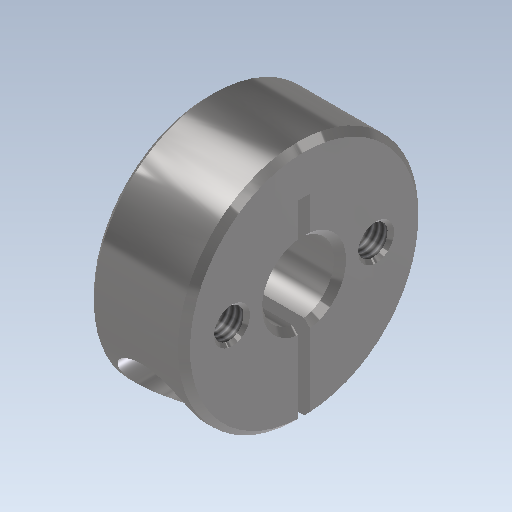
# Autodesk Inventor part: SCSW6-8b
Saved by Autodesk Inventor 2021 (Build 250183000, 183)
## iProperties
Created: 2019-10-03
Part Number: SCSW6-8b
Material: 鋼、炭素鋼
Catalog Web Link: www.cadenas.de
Description: SCSW, PSCSW, SSCSW-b-Shaft Collars - 2 Holes/2 Taps - 2-Tapped (Coarse Thread)
Vendor: MISUMI
Document SubType Name: Modeling
Designer: psadmin
Manufacturer: MISUMI
Mass: 15.1833 g
Surface Area: 15.2751 cm^2
Volume: 1.93418 cm^3
Density: 7.85 g/cm^3
Appearance: 半つや出し
Category: PARTsolutions
Company: MISUMI
PSOL_IDENT_0: {$CADENAS_DATA\23d-libs\misumi\metric\03_set_collars\scsw_b.prj},182 {VTYP=3D},{NB=SCSW6-8b},{LINA=S
PSOL_IDENT_1: CSW6-8b},{NN=SCSW, PSCSW, SSCSW-b},{DATE=30.03.2018 01:14:49},{GEOMDATE=24.02.2016 04:36:42},{VERSIO
PSOL_IDENT_2: N=},{LINEID=220},{WBVAR=MAT,ST,BS},{WBNUMERIC=BS}  {NB=SCSW6-8b},{LINA=SCSW6-8b},{KT=DUMMY},{PN=SCSW
PSOL_IDENT_3: 6-8},{TYPE=SCSW},{MAT=1045},{ST=Black Oxide},{AC=Hexagon Socket Head Set Screw 1 Pc.},{D=6},{BS=8},{
PSOL_IDENT_4: D1=20},{M=M3},{THMD=3},{THDMIN=2.459},{ST0='Black Oxide','Black Oxide','Electroless Nickel Plating','
PSOL_IDENT_5: Electroless Nickel Plating'},{B1=8,10},{DD=3.4},{R=3.00},{W=1.0},{X=6.0},{Y=4.0},{Z=6~6.5},{S=3.5},{
PSOL_IDENT_6: P=12},{C=0.5},{L=10},{M1=M3},{ZZ=6.25},{THMD1=3},{THDMIN1=2.459}
NN: SCSW, PSCSW, SSCSW-b
NT: Shaft Collars - 2 Holes/2 Taps - 2-Tapped (Coarse Thread)
NB: SCSW6-8b
NBSYN: $PN.b
LINA: SCSW6-8b
PN: SCSW6-8
MAT: S45C Equivalent
ST: Black Oxide
AC: Hexagon Socket Head Set Screw 1 Pc.
D: 6
BS: 8
D1: 20
M: M3
DD: 3.4
R: 3
W: 1
X: 6
Y: 4
Z: 6~6.5
S: 3.5
P: 12
M1: M3
SUPPLIER: MISUMI
ARTICLENO: SCSW6-8b
BOMINFO: SCSW6-8b
CREATOR: CADENAS GmbH
d17: 0.000 mm
Title: SCSW6-8b
Author: Cadenas PARTsolutions
Comments: Shaft Collars - 2 Holes/2 Taps - 2-Tapped (Coarse Thread)
Autodesk Inventor part; units mm, degrees
sketch "Sketch_1" plane through (0, 0, 0) normal (0, 0, 1) x (1, 0, 0)
  line L0 (4, 0) -> (-4, 0)
  line L1 (-4, 9.5) -> (-4, 3.5)
  line L2 (-4, 3.5) -> (-3.5, 3)
  line L3 (-3.5, 3) -> (3.5, 3)
  line L4 (3.5, 3) -> (4, 3.5)
  line L5 (4, 3.5) -> (4, 9.5)
  line L6 (4, 9.5) -> (3.5, 10)
  line L7 (3.5, 10) -> (-3.5, 10)
  line L8 (-3.5, 10) -> (-4, 9.5)
  constraints: 18 end point
revolve "Revolution1" add sketch "Sketch_1" angle 360 about axis through (4, 0, 0) along (1, 0, 0)
sketch "Sketch_2" plane through (0, 0, 0) normal (1, 0, 0) x (0, 1, 0)
  line L0 (-10, 0.5) -> (-10, -0.5)
  line L1 (-10, -0.5) -> (6.25, -0.5)
  line L2 (6.25, -0.5) -> (6.25, 0.5)
  line L3 (6.25, 0.5) -> (-10, 0.5)
  constraints: 8 end point
extrude "Extrusion1" cut sketch "Sketch_2" along normal mid plane 8
sketch "Sketch_3" plane through (0, 0, 0) normal (1, 0, 0) x (0, 1, 0)
  line L0 (-6, 10) -> (-6, 0)
  line L1 (-6, 0) -> (-7.7, 0)
  line L2 (-7.7, 0) -> (-7.7, 4)
  line L3 (-7.7, 4) -> (-9, 4)
  line L4 (-9, 4) -> (-9, 10)
  line L5 (-9, 10) -> (-6, 10)
  line L6 (-6, 10) -> (-6, 0)
  constraints: 14 end point
revolve "Revolution2" cut sketch "Sketch_3" angle 360 about axis through (0, -6, 10) along (0, 0, 1)
sketch "Sketch4" plane through (-3.5, -2.958, -0.5) normal (0, 0, 1) x (1, 0, 0)
  point P0 (3.5, -3.042)
hole "Hole1" at (0, -6, -0.5) direction (0, 0, -1) diameter 2.459 depth 9 countersink diameter 3 countersink angle 90 thread size "M3x0.5" class "6H" standard "ISO Metric profile"
sketch "Sketch_7" plane through (0, 0, -6) normal (0, 0, 1) x (1, 0, 0)
  line L0 (4, 0) -> (-4, 0)
  line L1 (-4, 0) -> (-4, 1.5)
  line L2 (-4, 1.5) -> (-3.7295, 1.2295)
  line L3 (-3.7295, 1.2295) -> (3.7295, 1.2295)
  line L4 (3.7295, 1.2295) -> (4, 1.5)
  line L5 (4, 1.5) -> (4, 0)
  line L6 (4, 0) -> (-4, 0)
  constraints: 14 end point
revolve "Revolution3" cut sketch "Sketch_7" angle 360 about axis through (4, 0, -6) along (1, 0, 0)
thread "Thread1" size "M3x0.5" class "6H" standard "ISO Metric profile" full length
sketch "Sketch_8" plane through (0, 0, 6) normal (0, 0, 1) x (1, 0, 0)
  line L0 (4, 0) -> (-4, 0)
  line L1 (-4, 0) -> (-4, 1.5)
  line L2 (-4, 1.5) -> (-3.7295, 1.2295)
  line L3 (-3.7295, 1.2295) -> (3.7295, 1.2295)
  line L4 (3.7295, 1.2295) -> (4, 1.5)
  line L5 (4, 1.5) -> (4, 0)
  line L6 (4, 0) -> (-4, 0)
  constraints: 14 end point
revolve "Revolution4" cut sketch "Sketch_8" angle 360 about axis through (4, 0, 6) along (1, 0, 0)
thread "Thread2" size "M3x0.5" class "6H" standard "ISO Metric profile" full length
ref_plane "body_screw_XY" through (0, -6, 4) normal (0, 0, 1) x (1, 0, 0)
ref_plane "body_screw_YZ" through (0, -6, 4) normal (1, 0, 0) x (0, 1, 0)
ref_plane "body_screw_ZX" through (0, -6, 4) normal (0, 1, 0) x (0, 0, 1)
body "Solid1"
